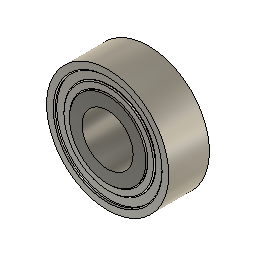
RollerBearing12x5x4 v3 (Autodesk Fusion 360 design; units mm, degrees)
Autodesk Fusion 360 part; units mm, degrees
sketch "Sketch1" plane through (0, 0, 0) normal (0, 1, 0) x (1, 0, 0)
  circle A0 centre (0, 0) radius 2.5
  circle A1 centre (0, 0) radius 3.75
  circle A2 centre (0, 0) radius 6
  circle A3 centre (0, 0) radius 5.25
  circle A4 centre (0, 0) radius 4.5
  dimension "d1" = 5
  dimension "d2" = 7.5
  dimension "d3" = 12
  dimension "d4" = 10.5
  dimension "d13" = 9
  constraint coincident A0.centre A1.centre
  constraint concentric A1 A2
  constraint concentric A1 A3
  constraint concentric A2 A4
  measures "d1" diameter of A0
  measures "d2" diameter of A1
  measures "d3" diameter of A2
  measures "d4" diameter of A3
  measures "d13" diameter of A4
extrude "Extrude1" add sketch "Sketch1" along normal blind 4 contours A2 | A3 | A4 makes body 1
extrude "Extrude2" add sketch "Sketch1" along normal blind 4 separate body contours A1 makes body 2
extrude "Extrude3" cut sketch "Sketch1" along normal blind 0.25 contours A3 bodies 1
sketch "Sketch2" plane through (0, 4, 0) normal (0, 1, 0) x (-1, 0, 0)
  circle A0 centre (0, 0) radius 3.75
  circle A1 centre (0, 0) radius 6
  circle A2 centre (0, 0) radius 5.25
  circle A3 centre (0, 0) radius 4.5
extrude "Extrude4" cut sketch "Sketch2" against normal blind 0.25 contours A2 bodies 1
extrude "Extrude5" cut 1 faces at (4.2193, 0, 0.4099) along direction (0, 1, 0) blind 0.1 on bodies 1 bodies 1
extrude "Extrude6" cut 1 faces at (-4.2193, 4, -0.4099) along direction (0, -1, 0) blind 0.1 on bodies 1 bodies 1
fillet "Fillet2" radius 0.1 6 edges at (-3.4962, 3.9, 1.3561) (4.1955, 3.9, 1.6273) (4.8947, 4, 1.8985) (-4.8947, 0, 1.8985) (-4.1955, 0.1, 1.6273) (-3.4962, 0.1, -1.3561) on bodies 1
